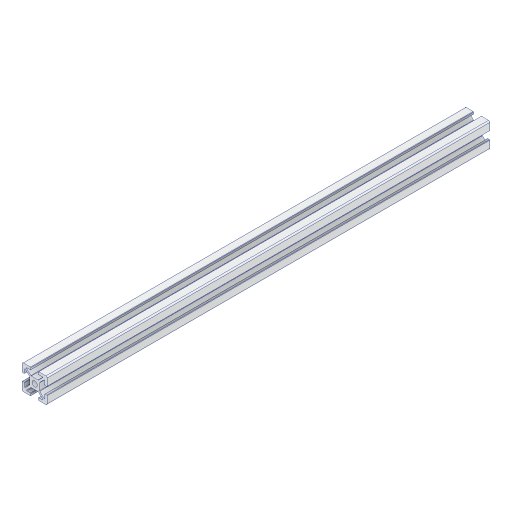
# Autodesk Inventor part: II Strebe senkrecht Türe
Saved by Autodesk Inventor 2023 (Build 270158000, 158)
## iProperties
Created: 2022-09-26
Part Number: II Strebe senkrecht Türe
Material: Aluminium 6061
Document SubType Name: Modeling
Designer: musati
Density: 2.7 g/cm^3
Appearance: Aluminum - Flat
Author: musati
Autodesk Inventor part; units mm, degrees
ref_plane "YZ Plane" through (0, 0, 0) normal (1, 0, 0) x (0, 1, 0)
ref_plane "XZ Plane" through (0, 0, 0) normal (0, 1, 0) x (-1, 0, 0)
ref_plane "XY Plane" through (0, 0, 0) normal (0, 0, 1) x (1, 0, 0)
sketch "Skizze1" plane through (0, 0, 0) normal (0, 0, 1) x (1, 0, 0)
  line L0 (-28.0083, 0) -> (28.0083, 0) projected
  line L1 (0, -28.0083) -> (0, 28.0083) projected
  line L2 (-14, 0) -> (14, 0)
  line L3 (0, -14) -> (0, 14)
  line L4 (-20.0059, 0) -> (20.0059, 0)
  line L5 (0, -20.0059) -> (0, 20.0059)
  line L6 (-14.2899, 0) -> (14.2899, 0)
  line L7 (0, -14.2899) -> (0, 14.2899)
  line L8 (-10, -10) -> (10, 10) construction
  line L9 (10, -10) -> (-10, 10) construction
  line L10 (-8, -8) -> (8, 8) construction
  line L11 (8, -8) -> (-8, 8) construction
  line L12 (-2.7322, -4) -> (2.7322, -4)
  line L13 (4, -2.7322) -> (4, 2.7322)
  line L14 (2.7322, 4) -> (-2.7322, 4)
  line L15 (-4, 2.7322) -> (-4, -2.7322)
  line L16 (-4, -4) -> (4, 4) construction
  line L17 (4, -4) -> (-4, 4) construction
  arc A0 (-9, 10) -> (-10, 9) centre (-9, 9) ccw
  arc A1 (10, 9) -> (9, 10) centre (9, 9) ccw
  arc A2 (9, -10) -> (10, -9) centre (9, -9) ccw
  arc A3 (-10, -9) -> (-9, -10) centre (-9, -9) ccw
  line L18 (-3, 9.7) -> (-3, 8.3)
  line L19 (3, 9.7) -> (3, 8.3)
  line L20 (6.2151, 8) -> (3.3, 8)
  line L21 (-3.3, 8) -> (-6.2151, 8)
  line L22 (9, 10) -> (3.3, 10)
  line L23 (-3.3, 10) -> (-9, 10)
  line L24 (-9.7, -3) -> (-8.3, -3)
  line L25 (-9.7, 3) -> (-8.3, 3)
  line L26 (-8, 6.2151) -> (-8, 3.3)
  line L27 (-8, -3.3) -> (-8, -6.2151)
  line L28 (-10, 9) -> (-10, 3.3)
  line L29 (-10, -3.3) -> (-10, -9)
  line L30 (-3, -8.3) -> (-3, -9.7)
  line L31 (3, -8.3) -> (3, -9.7)
  line L32 (-9, -10) -> (-3.3, -10)
  line L33 (3.3, -10) -> (9, -10)
  line L34 (-6.2151, -8) -> (-3.3, -8)
  line L35 (3.3, -8) -> (6.2151, -8)
  line L36 (8.3, 3) -> (9.7, 3)
  line L37 (8.3, -3) -> (9.7, -3)
  line L38 (8, -6.2151) -> (8, -3.3)
  line L39 (8, 3.3) -> (8, 6.2151)
  line L40 (10, -9) -> (10, -3.3)
  line L41 (10, 3.3) -> (10, 9)
  arc A4 (-10, 3.3) -> (-9.7, 3) centre (-9.7, 3.3) ccw
  arc A5 (-8.3, 3) -> (-8, 3.3) centre (-8.3, 3.3) ccw
  arc A6 (-9.7, -3) -> (-10, -3.3) centre (-9.7, -3.3) ccw
  arc A7 (-8, -3.3) -> (-8.3, -3) centre (-8.3, -3.3) ccw
  arc A8 (-3.3, -10) -> (-3, -9.7) centre (-3.3, -9.7) ccw
  arc A9 (-3, -8.3) -> (-3.3, -8) centre (-3.3, -8.3) ccw
  arc A10 (3, -9.7) -> (3.3, -10) centre (3.3, -9.7) ccw
  arc A11 (3.3, -8) -> (3, -8.3) centre (3.3, -8.3) ccw
  arc A12 (8.3, -3) -> (8, -3.3) centre (8.3, -3.3) ccw
  arc A13 (10, -3.3) -> (9.7, -3) centre (9.7, -3.3) ccw
  arc A14 (8, 3.3) -> (8.3, 3) centre (8.3, 3.3) ccw
  arc A15 (9.7, 3) -> (10, 3.3) centre (9.7, 3.3) ccw
  arc A16 (3, 8.3) -> (3.3, 8) centre (3.3, 8.3) ccw
  arc A17 (3.3, 10) -> (3, 9.7) centre (3.3, 9.7) ccw
  arc A18 (-3.3, 8) -> (-3, 8.3) centre (-3.3, 8.3) ccw
  arc A19 (-3, 9.7) -> (-3.3, 10) centre (-3.3, 9.7) ccw
  line L42 (-7.4879, 6.4272) -> (-4.1464, 3.0858)
  line L43 (-6.4272, 7.4879) -> (-3.0858, 4.1464)
  line L44 (-6.4272, -7.4879) -> (-3.0858, -4.1464)
  line L45 (-7.4879, -6.4272) -> (-4.1464, -3.0858)
  arc A20 (-7.4879, 6.4272) -> (-8, 6.2151) centre (-7.7, 6.2151) ccw
  arc A21 (-6.2151, 8) -> (-6.4272, 7.4879) centre (-6.2151, 7.7) ccw
  arc A22 (-8, -6.2151) -> (-7.4879, -6.4272) centre (-7.7, -6.2151) ccw
  arc A23 (-6.4272, -7.4879) -> (-6.2151, -8) centre (-6.2151, -7.7) ccw
  line L46 (6.4272, -7.4879) -> (3.0858, -4.1464)
  line L47 (4.1464, -3.0858) -> (7.4879, -6.4272)
  arc A24 (6.2151, -8) -> (6.4272, -7.4879) centre (6.2151, -7.7) ccw
  arc A25 (7.4879, -6.4272) -> (8, -6.2151) centre (7.7, -6.2151) ccw
  line L48 (4.1464, 3.0858) -> (7.4879, 6.4272)
  line L49 (3.0858, 4.1464) -> (6.4272, 7.4879)
  arc A26 (6.4272, 7.4879) -> (6.2151, 8) centre (6.2151, 7.7) ccw
  arc A27 (8, 6.2151) -> (7.4879, 6.4272) centre (7.7, 6.2151) ccw
  arc A28 (-3.0858, 4.1464) -> (-2.7322, 4) centre (-2.7322, 4.5) ccw
  arc A29 (-4, 2.7322) -> (-4.1464, 3.0858) centre (-4.5, 2.7322) ccw
  arc A30 (2.7322, 4) -> (3.0858, 4.1464) centre (2.7322, 4.5) ccw
  arc A31 (4.1464, 3.0858) -> (4, 2.7322) centre (4.5, 2.7322) ccw
  arc A32 (-4.1464, -3.0858) -> (-4, -2.7322) centre (-4.5, -2.7322) ccw
  arc A33 (-2.7322, -4) -> (-3.0858, -4.1464) centre (-2.7322, -4.5) ccw
  arc A34 (3.0858, -4.1464) -> (2.7322, -4) centre (2.7322, -4.5) ccw
  arc A35 (4, -2.7322) -> (4.1464, -3.0858) centre (4.5, -2.7322) ccw
  circle A36 centre (0, 0) radius 2.1
  point P0 (-3, 9.1415)
  point P1 (3, 8.9014)
  point P2 (-8.9764, -3)
  point P3 (-9.1265, 3)
  point P4 (-3, -9.1251)
  point P5 (3, -9.1251)
  point P6 (9.1101, 3)
  point P7 (9.1101, -3)
  dimension "d0" = 20
  dimension "d1" = 20
  dimension "d2" = 16
  dimension "d3" = 16
  dimension "d4" = 8
  dimension "d5" = 8
  dimension "d6" = 1
  dimension "d7" = 6
  dimension "d8" = 6
  dimension "d9" = 6
  dimension "d10" = 6
  dimension "d11" = 0.3
  dimension "d12" = 1.5
  dimension "d13" = 1.5
  dimension "d14" = 0.3
  dimension "d15" = 1.5
  dimension "d16" = 0.3
  dimension "d17" = 1.5
  dimension "d18" = 0.3
  dimension "d19" = 0.5
  dimension "d20" = 4.2
  dimension "d21" = 45
  dimension "d22" = 10
  dimension "d23" = 10
  dimension "d24" = 4
  dimension "d25" = 4
  dimension "d26" = 10
  dimension "d27" = 8
  dimension "d28" = 4
  dimension "d29" = 4
  dimension "d30" = 10
  dimension "d31" = 9.1101
  dimension "d32" = 8
  dimension "d33" = 4
  dimension "d34" = 8.9014
  dimension "d35" = 9.1251
  dimension "d36" = 9.1415
  dimension "d37" = 8.9764
  dimension "d38" = 9.1265
  constraints: 96 end point, 90 tangent, 72 point on circle, 37 centre point, 30 equal radius, 23 parallel, 15 perpendicular, 8 point on line, 7 horizontal, 6 midpoint, 2 vertical, 1 coincident, 8 other
  measures "d0" distance of L9.end L8.end
  measures "d1" distance of L8.end L9.start
  measures "d2" distance of L11.end L10.end
  measures "d3" distance of L10.end L11.start
  measures "d4" distance of L17.end L16.end
  measures "d5" distance of L16.end L17.start
  measures "d6" radius of A0
  measures "d7" horizontal distance of point (3, 8.901) point (-3, 9.142)
  measures "d8" vertical distance of point (-8.976, -3) point (-9.127, 3)
  measures "d9" distance of point (3, -9.125) point (-3, -9.125)
  measures "d10" distance of point (9.11, -3) point (9.11, 3)
  measures "d11" radius of A4
  measures "d12" distance between parallel lines of L43 L42
  measures "d13" distance between parallel lines of L45 L44
  measures "d14" radius of A20
  measures "d15" distance between parallel lines of L46 L47
  measures "d16" radius of A24
  measures "d17" distance between parallel lines of L49 L48
  measures "d18" radius of A26
  measures "d19" radius of A28
  measures "d20" diameter of A36
  measures "d21" angle of L47 L7
  measures "d22" distance between parallel lines of L41 L7
  measures "d23" distance between parallel lines of L22 L6
  measures "d24" distance between parallel lines of L12 L6
  measures "d25" distance between parallel lines of L15 L7
  measures "d26" distance between parallel lines of L29 L7
  measures "d27" distance between parallel lines of L34 L6
  measures "d28" distance between parallel lines of L13 L7
  measures "d29" distance between parallel lines of L14 L6
  measures "d30" distance from line of L8.end L7
  measures "d31" distance from line of point (9.11, 3) L7
  measures "d32" distance from line of L10.end L7
  measures "d33" distance from line of L16.end L7
  measures "d34" distance from line of point (3, 8.901) L6
  measures "d35" distance from line of point (3, -9.125) L6
  measures "d36" distance from line of point (-3, 9.142) L6
  measures "d37" distance from line of point (-8.976, -3) L7
  measures "d38" distance from line of point (-9.127, 3) L7
extrude "Extrusion1" add sketch "Skizze1" against normal blind 355 contours L15 A29 L42 A20 L26 A5 L25 A4 L28 A0 L23 A19 L18 A18 L21 A21 L43 A28 L14 L1 A36 L0 | L0 A36 L1 L12 A33 L44 A23 L34 A9 L30 A8 L32 A3 L29 A6 L24 A7 L27 A22 L45 A32 L15 | L1 L14 A30 L49 A26 L20 A16 L19 A17 L22 A1 L41 A15 L36 A14 L39 A27 L48 A31 L13 L0 A36 | A36 L0 L13 A35 L47 A25 L38 A12 L37 A13 L40 A2 L33 A10 L31 A11 L35 A24 L46 A34 L12 L1
